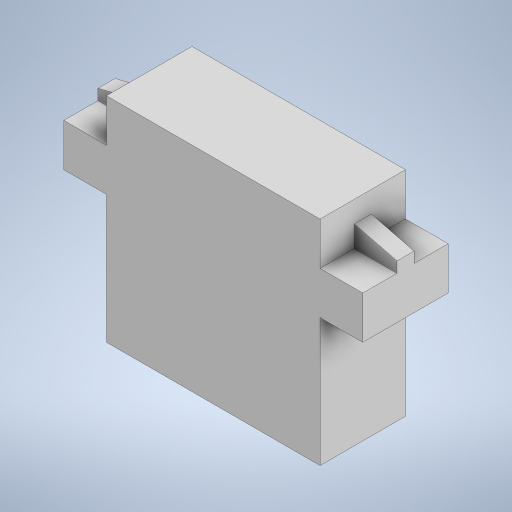
# Autodesk Inventor part: Servomotor
Saved by Autodesk Inventor 2023 (Build 270158000, 158)
## iProperties
Created: 2023-07-27
Part Number: Servomotor
Material: Generic
Document SubType Name: Modeling
Designer: User
Density: 1 g/cm^3
Appearance: Default
Author: User
Autodesk Inventor part; units mm, degrees
ref_plane "YZ Plane" through (0, 0, 0) normal (1, 0, 0) x (0, 1, 0)
ref_plane "XZ Plane" through (0, 0, 0) normal (0, 1, 0) x (-1, 0, 0)
sketch "Sketch1" plane through (0, 0, 0) normal (0, 0, 1) x (1, 0, 0)
  line L0 (0, 0) -> (-25, 0)
  line L1 (-25, 0) -> (-25, 50)
  line L2 (-25, 50) -> (0, 50)
  line L3 (0, 50) -> (0, 0)
  line L4 (-25, 30) -> (-35, 30)
  line L5 (-35, 30) -> (-35, 40)
  line L6 (-35, 40) -> (-25, 40)
  line L7 (-25, 40) -> (-25, 30)
  line L8 (0, 0) -> (25, 0)
  line L9 (25, 0) -> (25, 50)
  line L10 (25, 50) -> (0, 50)
  line L11 (25, 30) -> (35, 30)
  line L12 (35, 30) -> (35, 40)
  line L13 (35, 40) -> (25, 40)
  dimension "d0" = 25
  dimension "d1" = 50
  dimension "d2" = 30
  dimension "d3" = 10
  dimension "d4" = 10
  constraints: 28 end point, 6 symmetric about line, 4 parallel, 2 horizontal, 2 perpendicular, 2 point on line
  measures "d0" distance of L1.end L2.end
  measures "d1" distance of L0.end L1.end
  measures "d2" distance from line of L4 L0.end
  measures "d3" distance of L6.end L4.start
  measures "d4" distance of L4.start L4.end
extrude "Extrusion1" add sketch "Sketch1" along normal mid plane 20
ref_plane "Work Plane1" through (0, 0, 0) normal (0, 0, 1) x (1, 0, 0)
sketch "Sketch2" plane through (0, 0, 0) normal (0, 0, 1) x (1, 0, 0)
  line L0 (-25, 50) -> (-25, 40) projected
  line L1 (-25, 40) -> (-35, 40)
  line L2 (-35, 40) -> (-35, 42.5)
  line L3 (-25, 45) -> (-25, 40)
  line L4 (-25, 42.5) -> (-25, 45)
  line L5 (-25, 45) -> (-35, 42.5)
  line L6 (0, 0) -> (0, 50)
  line L7 (25, 50) -> (-25, 50) projected
  line L8 (25, 45) -> (25, 40)
  line L9 (25, 40) -> (35, 40)
  line L10 (35, 40) -> (35, 42.5)
  line L11 (25, 45) -> (35, 42.5)
  constraints: 20 end point, 4 symmetric about line, 1 horizontal, 1 midpoint, 1 parallel, 1 perpendicular
extrude "Extrusion2" add sketch "Sketch2" along normal mid plane 4
body "Solid1"
